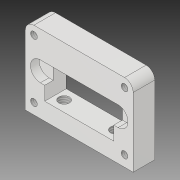
# Autodesk Inventor part: Kamerahalter Vorne
Saved by Autodesk Inventor 2019.1 (Build 231200000, 200)
## iProperties
Part Number: Kamerahalter Vorne
Material: PC/ABS-Kunststoff
Document SubType Name: Modeling
Designer: rYan
Mass: 0.532056 g
Surface Area: 14.5072 cm^2
Volume: 1.48921 cm^3
Density: 0.357273 g/cm^3
Appearance: Glatt - Weiß
Author: rYan
Autodesk Inventor part; units mm, degrees
ref_plane "YZ Plane" through (0, 0, 0) normal (1, 0, 0) x (0, 1, 0)
ref_plane "XZ Plane" through (0, 0, 0) normal (0, 1, 0) x (-1, 0, 0)
ref_plane "XY Plane" through (0, 0, 0) normal (0, 0, 1) x (1, 0, 0)
sketch "Skizze1" plane through (0, 0, 0) normal (0, 1, 0) x (-1, 0, 0)
  line L0 (12.5, -9) -> (-12.5, -9)
  line L1 (-12.5, -9) -> (-12.5, 9)
  line L2 (-12.5, 9) -> (12.5, 9)
  line L3 (12.5, 9) -> (12.5, -9)
  line L4 (12.5, -9) -> (-12.5, 9) construction
  line L5 (-12.5, -9) -> (12.5, 9) construction
  line L6 (8, -5) -> (-8, -5)
  line L7 (-8, -5) -> (-8, 2.8)
  line L8 (-8, 2.8) -> (8, 2.8)
  line L9 (8, 2.8) -> (8, -5)
  line L10 (0, 2.8) -> (0, -5) construction
  point P0 (0, 0)
  point P1 (0, 0)
  dimension "d0" = 25
  dimension "d1" = 18
  dimension "d23" = 16
  dimension "d28" = 4
  dimension "d29" = 7.8
  constraints: 22 end point, 5 midpoint, 4 parallel, 2 horizontal, 2 perpendicular, 1 point on line
  measures "d0" distance of L1.end L2.end
  measures "d1" distance of L0.end L1.end
  measures "d23" distance of L7.end L8.end
  measures "d28" distance between parallel lines of L6 L0
  measures "d29" distance of L6.end L7.end
extrude "Extrusion1" add sketch "Skizze1" along normal mid plane 5
sketch "Skizze2" plane through (0, -2.5, 0) normal (0, -1, 0) x (1, 0, 0)
  line L0 (-10.5, 7) -> (10.5, 7) construction
  line L1 (10.5, 7) -> (10.5, -6.5) construction
  line L2 (10.5, -6.5) -> (-10.5, -6.5) construction
  line L3 (-10.5, -6.5) -> (-10.5, 7) construction
  line L4 (0, 12.6) -> (0, -12.6) projected
  line L5 (12.5, 9) -> (-12.5, 9) projected
  point P0 (0, 0)
  dimension "d4" = 21
  dimension "d5" = 13.5
  dimension "d6" = 2
  constraints: 8 end point, 4 coincident, 2 parallel, 1 horizontal, 1 perpendicular, 1 other
  measures "d4" distance of L0.start L0.end
  measures "d5" distance of L0.end L1.end
  measures "d6" distance between parallel lines of L5 L0
hole "Bohrung1" at (-10.5, -2.5, 7) at (10.5, -2.5, 7) at (10.5, -2.5, -6.5) at (-10.5, -2.5, -6.5) direction (0, 1, 0) diameter 1.567 end through all thread size "M2x0.4" class "6H" standard "ISO Metric profile"
sketch "Skizze3" plane through (12.5, 2.5, -9) normal (0, 0, -1) x (-1, 0, 0)
  line L0 (25, -5) -> (25, 0) projected
  line L1 (0, 0) -> (25, 0) projected
  line L2 (0, 0) -> (0, -5) projected
  line L3 (25, -5) -> (0, -5) projected
  line L4 (25, -2.5) -> (0, -2.5) construction
  line L5 (0, -5) -> (25, -5) construction
  line L6 (12.5, -5) -> (12.5, 0) construction
  line L7 (25, 0) -> (0, 0) construction
  point P0 (12.5, -2.5)
  point P1 (18.5, -2.5)
  point P2 (6.5, -2.5)
  dimension "d14" = 12
  constraints: 4 end point, 4 midpoint, 2 point on line, 1 symmetric about line
  measures "d14" distance of point (6.5, -2.5) point (18.5, -2.5)
hole "Bohrung2" at (-6, 0, -9) at (6, 0, -9) direction (0, 0, 1) diameter 2.459 depth 4 thread size "M3x0.5" class "6H" standard "ISO Metric profile"
fillet "Rundung1" radius 2 2 edges at (-12.5, 0, 9) (12.5, 0, 9)
sketch "Skizze4" plane through (0, -2.5, 0) normal (0, -1, 0) x (1, 0, 0)
  line L0 (-9, 0.5) -> (9, 0.5) construction
  line L1 (-9, -1.8) -> (9, -1.8)
  line L2 (9, 2.8) -> (-9, 2.8)
  arc A0 (-9, 2.8) -> (-9, -1.8) centre (-9, 0.5) ccw
  arc A1 (9, -1.8) -> (9, 2.8) centre (9, 0.5) ccw
  line L3 (0, 12.6) -> (0, -12.6) projected
  line L4 (-12.5, -9) -> (12.5, -9) projected
  point P0 (0, 0)
  point P1 (0, 0.5)
  dimension "d24" = 4.6
  dimension "d25" = 18
  dimension "d30" = 9.5
  constraints: 8 end point, 4 point on circle, 4 tangent, 2 centre point, 1 horizontal, 1 midpoint, 1 parallel, 1 point on line
  measures "d24" diameter of A1
  measures "d25" distance of L0.start L0.end
  measures "d30" distance between parallel lines of L0 L4
extrude "Extrusion2" cut sketch "Skizze4" against normal blind 2
